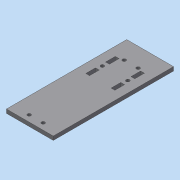
# Autodesk Inventor part: bed-axis
Saved by Autodesk Inventor 2016 SP1 (Build 200210100, 210)
## iProperties
Created: 2016-03-25
Part Number: bed-axis
Material: Generic
Document SubType Name: Modeling
Designer: Mohamed A.
Density: 1 g/cm^3
Appearance: Default
Author: Mohamed A.
Autodesk Inventor part; units mm, degrees
ref_plane "YZ Plane" through (0, 0, 0) normal (1, 0, 0) x (0, 1, 0)
ref_plane "XZ Plane" through (0, 0, 0) normal (0, 1, 0) x (-1, 0, 0)
ref_plane "XY Plane" through (0, 0, 0) normal (0, 0, 1) x (1, 0, 0)
sketch "Sketch1" plane through (0, 0, 0) normal (0, 0, 1) x (1, 0, 0)
  line L0 (-18.5, 78.1667) -> (18.5, 78.1667)
  line L1 (18.5, 78.1667) -> (18.5, -41.8333)
  line L2 (-18.5, -41.8333) -> (-18.5, 78.1667)
  line L3 (-18.5, 78.1667) -> (18.5, -41.8333) construction
  line L4 (18.5, 78.1667) -> (-18.5, -41.8333) construction
  line L5 (0, -66.8333) -> (0, 108.1667) construction
  line L6 (5.5, 68.1667) -> (-5.5, 68.1667) construction
  line L7 (-5.5, 68.1667) -> (-5.5, -36.8333) construction
  line L8 (-5.5, -36.8333) -> (5.5, -36.8333) construction
  line L9 (5.5, -36.8333) -> (5.5, 68.1667) construction
  circle A0 centre (-5.5, 68.1667) radius 1.35
  circle A1 centre (5.5, 68.1667) radius 1.35
  circle A2 centre (-5.5, -36.8333) radius 1.35
  circle A3 centre (5.5, -36.8333) radius 1.35
  line L10 (18.5, 78.1667) -> (-18.5, 78.1667)
  line L11 (-18.5, 78.1667) -> (-18.5, 83.1667)
  line L12 (-18.5, 83.1667) -> (18.5, 83.1667)
  line L13 (18.5, 83.1667) -> (18.5, 78.1667)
  line L14 (-11.5, 59.5) -> (-8.5, 51.5) construction
  line L15 (-11.5, 51.5) -> (-8.5, 59.5) construction
  line L16 (11.5, 51.5) -> (8.5, 59.5) construction
  line L17 (8.5, 51.5) -> (11.5, 59.5) construction
  circle A4 centre (-10, 55.5) radius 1.35
  circle A5 centre (10, 55.5) radius 1.35
  line L18 (-8.5, 67.1667) -> (-8.5, 59.5) projected
  line L19 (-8.5, 67.1667) -> (-11.5, 67.1667) projected
  line L20 (-11.5, 59.5) -> (-11.5, 67.1667) projected
  line L21 (-8.5, 59.5) -> (-11.5, 59.5) projected
  line L22 (11.5, 51.5) -> (11.5, 43.8333) projected
  line L23 (11.5, 51.5) -> (8.5, 51.5) projected
  line L24 (8.5, 43.8333) -> (8.5, 51.5) projected
  line L25 (11.5, 43.8333) -> (8.5, 43.8333) projected
  line L26 (11.5, 67.1667) -> (11.5, 59.5) projected
  line L27 (11.5, 67.1667) -> (8.5, 67.1667) projected
  line L28 (8.5, 59.5) -> (8.5, 67.1667) projected
  line L29 (11.5, 59.5) -> (8.5, 59.5) projected
  line L30 (-8.5, 51.5) -> (-8.5, 43.8333) projected
  line L31 (-8.5, 51.5) -> (-11.5, 51.5) projected
  line L32 (-11.5, 43.8333) -> (-11.5, 51.5) projected
  line L33 (-8.5, 43.8333) -> (-11.5, 43.8333) projected
  line L34 (18.5, -41.8333) -> (-18.5, -41.8333)
  point P0 (0, 0)
  point P1 (0, 18.1667)
  point P2 (0, 18.1667)
  dimension "d1" = 37
  dimension "d4" = 11
  dimension "d6" = 2.7
  dimension "d7" = 2.7
  dimension "d8" = 2.7
  dimension "d9" = 2.7
  dimension "d11" = 2.7
  dimension "d12" = 2.7
  dimension "d14" = 13
  dimension "d15" = 1
  dimension "d18" = 120
  constraints: 36 end point, 7 parallel, 6 centre point, 5 horizontal, 5 midpoint, 4 coincident, 4 perpendicular, 1 point on line
  measures "d1" distance of L1.end L2.start
  measures "d4" distance between parallel lines of L9 L7
  measures "d6" diameter of A0
  measures "d7" diameter of A1
  measures "d8" diameter of A2
  measures "d9" diameter of A3
  measures "d11" diameter of A4
  measures "d12" diameter of A5
  measures "d14" distance between parallel lines of L2 L7
  measures "d15" distance between parallel lines of L6 L19
  measures "d18" distance between parallel lines of L34 L0
extrude "Extrusion1" add sketch "Sketch1" along normal blind 3
body "Solid1"
